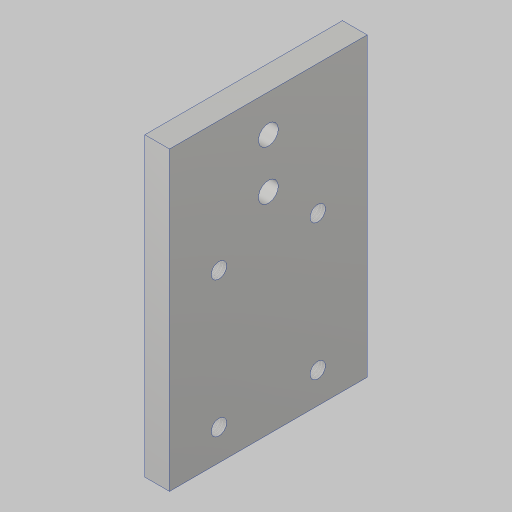
# Autodesk Inventor part: EL2-027
Saved by Autodesk Inventor 2023.5 (Build 275446000, 446)
## iProperties
Created: 2025-02-12
Part Number: EL2-027
Material: Aluminum 6061
Document SubType Name: Modeling
Designer: slick
Density: 2.7 g/cm^3
Appearance: Aluminum - Flat
Author: slick
Autodesk Inventor part; units mm, degrees
ref_plane "YZ Plane" through (0, 0, 0) normal (1, 0, 0) x (0, 1, 0)
ref_plane "XZ Plane" through (0, 0, 0) normal (0, 1, 0) x (-1, 0, 0)
ref_plane "XY Plane" through (0, 0, 0) normal (0, 0, 1) x (1, 0, 0)
sketch "Sketch1" plane through (0, 0, 0) normal (1, 0, 0) x (0, 1, 0)
  line L0 (-38.1, -25.4) -> (38.1, -25.4)
  line L1 (38.1, -25.4) -> (38.1, 25.4)
  line L2 (38.1, 25.4) -> (-38.1, 25.4)
  line L3 (-38.1, 25.4) -> (-38.1, -25.4)
  line L4 (-38.1, -25.4) -> (38.1, 25.4) construction
  line L5 (38.1, -25.4) -> (-38.1, 25.4) construction
  point P0 (0, 0)
  dimension "d0" = 76.2
  dimension "d1" = 50.8
  constraints: 12 end point, 2 midpoint, 2 parallel, 1 horizontal, 1 perpendicular
  measures "d0" distance of L2.end L1.end
  measures "d1" distance of L1.end L0.end
extrude "Extrusion1" add sketch "Sketch1" along normal blind 6.35
sketch "Sketch2" plane through (6.35, 0, 0) normal (1, 0, 0) x (0, 0, -1)
  line L0 (12.7, -30.1498) -> (-12.7, -30.1498) construction
  line L1 (-12.7, -30.1498) -> (-12.7, 4.7752) construction
  line L2 (-12.7, 4.7752) -> (12.7, 4.7752) construction
  line L3 (12.7, 4.7752) -> (12.7, -30.1498) construction
  line L4 (12.7, -30.1498) -> (-12.7, 4.7752) construction
  line L5 (-12.7, -30.1498) -> (12.7, 4.7752) construction
  line L6 (-25.4, -38.1) -> (25.4, -38.1) construction
  line L7 (25.4, 38.1) -> (-25.4, 38.1) construction
  point P0 (0, 0)
  point P1 (0, -12.6873)
  point P2 (0, 28.575)
  point P3 (0, 15.875)
  point P4 (0, 38.1)
  point P5 (0, 38.1)
  dimension "d4" = 25.4
  dimension "d5" = 34.925
  dimension "d6" = 7.9502
  dimension "d7" = 12.7
  dimension "d8" = 9.525
  constraints: 12 end point, 4 coincident, 4 midpoint, 3 vertical alignment, 2 parallel, 1 horizontal, 1 perpendicular
  measures "d4" distance of L1.end L2.end
  measures "d5" distance of L0.end L1.end
  measures "d6" distance between parallel lines of L6 L0
  measures "d7" distance of point (0, 15.875) point (0, 28.575)
  measures "d8" distance of point (0, 38.1) point (0, 28.575)
hole "Hole1" at (6.35, -30.1498, 12.7) at (6.35, -30.1498, -12.7) at (6.35, 4.7752, -12.7) at (6.35, 4.7752, 12.7) direction (-1, 0, 0) diameter 3.9624 end through all thread size "10-32 UNF" class "2B" standard "ANSI Unified Screw Threads"
hole "Hole2" at (6.35, 28.575, 0) at (6.35, 15.875, 0) direction (-1, 0, 0) diameter 5.1054 end through all clearance for "Flat Head Machine Screw (82)" size "#10" standard "Ansi Unified Screw Threads"
body "Solid1"
